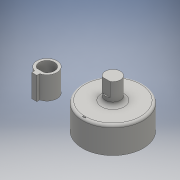
# Autodesk Inventor part: sprag_fill
Saved by Autodesk Inventor 2016 (Build 200138000, 138)
## iProperties
Created: 2017-07-02
Part Number: sprag_fill
Material: Generic
Document SubType Name: Modeling
Designer: ALIREZA
Density: 1 g/cm^3
Appearance: Default
Author: ALIREZA
Autodesk Inventor part; units mm, degrees
ref_plane "YZ Plane" through (0, 0, 0) normal (1, 0, 0) x (0, 1, 0)
ref_plane "XZ Plane" through (0, 0, 0) normal (0, 1, 0) x (-1, 0, 0)
ref_plane "XY Plane" through (0, 0, 0) normal (0, 0, 1) x (1, 0, 0)
sketch "Sketch1" plane through (0, 0, 0) normal (0, 0, 1) x (1, 0, 0)
  circle A0 centre (0, 0) radius 11.5
  dimension "d0" = 23
  constraints: 1 centre point, 1 coincident
  measures "d0" diameter of A0
sketch "Sketch2" plane through (0, 0, 0) normal (0, 0, 1) x (1, 0, 0)
  circle A0 centre (0, 0) radius 12
  dimension "d1" = 24
  constraints: 1 centre point, 1 coincident
  measures "d1" diameter of A0
extrude "Extrusion1" add sketch "Sketch2" along normal blind 10.5
extrude "Extrusion2" cut sketch "Sketch1" along normal blind 9
fillet "Fillet1" radius 0.5 1 edges at (-11.5, 0, 9)
sketch "Sketch3" plane through (0, 0, 10.5) normal (0, 0, 1) x (1, 0, 0)
  circle A0 centre (0, 0) radius 3
  dimension "d7" = 6
  constraints: 1 centre point, 1 coincident
  measures "d7" diameter of A0
extrude "Extrusion3" add sketch "Sketch3" along normal blind 8.5
fillet "Fillet2" radius 1 1 edges at (-12, 0, 10.5)
fillet "Fillet3" radius 1.5 1 edges at (-3, 0, 10.5)
sketch "Sketch4" plane through (0, 0, 19) normal (0, 0, 1) x (1, 0, 0)
  arc A0 (-1.5, -2.5981) -> (1.5154, -2.5891) centre (0, 0) ccw
  line L0 (-1.5, -2.5981) -> (1.5154, -2.5891)
  circle A1 centre (0, 0) radius 3 projected
  constraints: 2 end point, 2 point on circle, 1 centre point, 2 other
extrude "Extrusion4" cut sketch "Sketch4" against normal blind 5.5 contours L0 A0
sketch "Sketch5" plane through (0, 0, 10.5) normal (0, 0, 1) x (1, 0, 0)
  point P0 (0, 0)
sketch "Sketch6" plane through (0, 0, 0) normal (0, 0, -1) x (-1, 0, 0)
  circle A0 centre (26.1184, 0) radius 4
  circle A1 centre (26.1184, 0) radius 3
  point P0 (0, 0)
  dimension "d17" = 8
  dimension "d18" = 6
  constraints: 2 centre point, 1 coincident
  measures "d17" diameter of A0
  measures "d18" diameter of A1
extrude "Extrusion5" add sketch "Sketch6" against normal blind 9
sketch "Sketch7" plane through (-26.1184, 0, 0) normal (0, 0, -1) x (-1, 0, 0)
  circle A0 centre (0, 0) radius 3 projected
  line L0 (-1.5, -2.5981) -> (1.5, -2.5981)
  arc A1 (-1.5, -2.5981) -> (1.5, -2.5981) centre (0, 0) ccw
  circle A2 centre (0, 0) radius 4 projected
  line L1 (0, 0) -> (-1, 0)
  line L2 (0, -4) -> (0, -5)
  line L3 (0, -5) -> (-1, -5)
  line L4 (0, -5) -> (1, -5)
  line L5 (0, 0) -> (1, 0)
  line L6 (1, -3.873) -> (1, -5)
  line L7 (-1, -4.7888) -> (-1, -5)
  line L8 (-1, -3.873) -> (-1, -4.7888)
  line L9 (-1, -4.7888) -> (-1, -5)
  point P0 (-26.1184, 0)
  dimension "d22" = 1
  dimension "d23" = 1
  dimension "d24" = 1
  constraints: 20 end point, 7 point on circle, 3 horizontal, 3 perpendicular, 1 centre point, 1 concentric, 1 parallel, 1 vertical
  measures "d22" distance of L1.start L1.end
  measures "d23" distance of L2.start L2.end
  measures "d24" distance of L1.start L5.end
extrude "Extrusion6" add sketch "Sketch7" against normal up to surface (9 mm away) contours L0 A0 | A2 L2 L3 L7 L8 | L6 L4 L2 A2 picked at (-0.309, -2.6831)
sketch "Sketch8" plane through (0, 0, 0) normal (0, 0, -1) x (-1, 0, 0)
  circle A0 centre (0, 0) radius 11.5 projected
  line L0 (0.0233, -11.1929) -> (-0.4767, -11.1929)
  line L1 (-0.4767, -11.1929) -> (-0.4767, -11.4901)
  line L2 (0.0233, -11.1929) -> (0.5233, -11.1929)
  line L3 (0.5233, -11.1929) -> (0.5233, -11.4881)
  dimension "d27" = 0.5
  dimension "d28" = 0.5
  constraints: 8 end point, 2 perpendicular, 2 point on circle, 1 horizontal
  measures "d27" distance of L0.start L0.end
  measures "d28" distance of L0.start L2.end
extrude "Extrusion7" add sketch "Sketch8" against normal up to surface (10.5 mm away) contours L1 L0 L2 L3 A0 picked at (-0.1989, -11.295)
body "Solid1"
